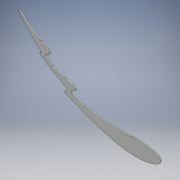
# Autodesk Inventor part: bracket
Saved by Autodesk Inventor 2018.2 (Build 222227000, 227)
## iProperties
Created: 2018-03-14
Part Number: bracket
Material: 一般
Document SubType Name: Modeling
Designer: ku_sk
Density: 1 g/cm^3
Appearance: 既定
Author: ku_sk
Autodesk Inventor part; units mm, degrees
ref_plane "YZ Plane" through (0, 0, 0) normal (1, 0, 0) x (0, 1, 0)
ref_plane "XZ Plane" through (0, 0, 0) normal (0, 1, 0) x (-1, 0, 0)
ref_plane "XY Plane" through (0, 0, 0) normal (0, 0, 1) x (1, 0, 0)
sketch "スケッチ1" plane through (0, 0, 0) normal (0, 1, 0) x (-1, 0, 0)
  arc A0 (352.9404, 45.4012) -> (350.2664, 52.9074) centre (351.268, 49.0348) ccw projected
  arc A1 (196.042, -12.8796) -> (352.9404, 45.4012) centre (-109.7603, 1050.7077) ccw projected
  arc A2 (150.312, -24.5744) -> (196.042, -12.8796) centre (-24.3171, 753.5344) ccw projected
  arc A3 (62.5903, -32.1265) -> (150.312, -24.5744) centre (78.6271, 294.8376) ccw projected
  arc A4 (7.8921, -21.3368) -> (62.5903, -32.1265) centre (71.9931, 159.5809) ccw projected
  arc A5 (-9.4003, -11.6891) -> (7.8921, -21.3368) centre (27.6212, 34.3463) ccw projected
  arc A6 (-8.119, 12.6128) -> (-9.4003, -11.6891) centre (0, 0) ccw projected
  arc A7 (11.7348, 20.8189) -> (-8.119, 12.6128) centre (24.3569, -37.8384) ccw projected
  arc A8 (90.7942, 27.108) -> (11.7348, 20.8189) centre (74.8452, -272.4677) ccw projected
  arc A9 (90.7942, 27.108) -> (95.7842, 26.8528) centre (154.5899, 1225.411) ccw projected
  arc A10 (95.7842, 26.8528) -> (350.2664, 52.9074) centre (137.4382, 875.8316) ccw projected
  arc A11 (451.6654, 129.0808) -> (449.8552, 131.7041) centre (450.6431, 130.3115) ccw projected
  arc A12 (397.0782, 90.3195) -> (451.6654, 129.0808) centre (168.8146, 469.5991) ccw projected
  arc A13 (380.6202, 81.0666) -> (397.0782, 90.3195) centre (232.593, 363.6259) ccw projected
  arc A14 (347.509, 69.0671) -> (380.6202, 81.0666) centre (319.8553, 197.0566) ccw projected
  arc A15 (325.2582, 67.5731) -> (347.509, 69.0671) centre (331.295, 144.1106) ccw projected
  arc A16 (317.5781, 69.5105) -> (325.2582, 67.5731) centre (327.1162, 91.13) ccw projected
  arc A17 (315.5573, 79.0327) -> (317.5781, 69.5105) centre (320, 75) ccw projected
  arc A18 (322.3786, 84.2587) -> (315.5573, 79.0327) centre (333.3281, 62.902) ccw projected
  arc A19 (352.2737, 94.8734) -> (322.3786, 84.2587) centre (377.1259, -22.5249) ccw projected
  arc A20 (352.2737, 94.8734) -> (354.2282, 95.2914) centre (252.865, 564.4668) ccw projected
  arc A21 (354.2282, 95.2914) -> (449.8552, 131.7041) centre (282.4293, 427.624) ccw projected
  arc A22 (533.1819, 231.3155) -> (533.0183, 233.3599) centre (531.8758, 232.2398) ccw projected
  arc A23 (490.4869, 179.7468) -> (533.1819, 231.3155) centre (171.8364, 487.0238) ccw projected
  arc A24 (476.9845, 166.5496) -> (490.4869, 179.7468) centre (260.8694, 401.1686) ccw projected
  arc A25 (448.1072, 146.3891) -> (476.9845, 166.5496) centre (388.2697, 262.8602) ccw projected
  arc A26 (427.0013, 139.1871) -> (448.1072, 146.3891) centre (413.023, 214.679) ccw projected
  arc A27 (419.0814, 139.0707) -> (427.0013, 139.1871) centre (422.699, 162.4222) ccw projected
  arc A28 (414.665, 147.7454) -> (419.0814, 139.0707) centre (420, 145) ccw projected
  arc A29 (419.9012, 154.5588) -> (414.665, 147.7454) centre (436.0051, 136.7638) ccw projected
  arc A30 (446.0304, 172.5493) -> (419.9012, 154.5588) centre (500.4207, 65.5835) ccw projected
  arc A31 (446.0304, 172.5493) -> (447.8101, 173.4589) centre (228.4693, 600.4128) ccw projected
  arc A32 (447.8101, 173.4589) -> (530.4702, 233.1021) centre (292.4437, 475.8846) ccw projected
  line L0 (530.4702, 233.1021) -> (525.5697, 238.1005) projected
  line L1 (525.5697, 238.1005) -> (526.9978, 239.5007) projected
  line L2 (526.9978, 239.5007) -> (533.0183, 233.3599) projected
  arc A33 (530.4702, 233.1021) -> (530.7544, 233.381) centre (292.4437, 475.8846) ccw
  arc A34 (533.0183, 233.3599) -> (530.7544, 233.381) centre (531.8758, 232.2398) ccw
  line L3 (317.5781, 69.5105) -> (338.9513, 60.0811)
  line L4 (338.9513, 60.0811) -> (283.0095, 38.3896)
  line L5 (380.6202, 81.0666) -> (345.1511, 62.485)
  line L6 (345.1511, 62.485) -> (354.3249, 51.6146)
  line L7 (419.0814, 139.0707) -> (435.7934, 136.4817)
  line L8 (435.7934, 136.4817) -> (395.4422, 106.9558)
  line L9 (476.9845, 166.5496) -> (443.1114, 135.348)
  line L10 (443.1114, 135.348) -> (451.2836, 131.7777)
  point P0 (0, 0)
  dimension "d2" = 45
  dimension "d3" = 45
  dimension "d4" = 60
  dimension "d5" = 50
  constraints: 16 end point, 8 point on circle, 7 tangent, 2 centre point, 2 concentric, 2 point on line
  measures "d2" angle of L4 L3
  measures "d3" angle of L8 L7
  measures "d4" distance of L3.end L4.end
  measures "d5" distance of L7.end L8.end
extrude "押し出し1" add sketch "スケッチ1" along normal mid plane 4 contours A1 A2 A3 A4 A5 A6 A7 A8 A9 A10 A0 | A0 A10 L4 L3 A16 A15 A14 L5 L6 | A14 A15 A16 A17 A18 A19 A20 A21 A11 A12 A13 | A11 A21 L8 L7 A27 A26 A25 L9 L10 | A25 A26 A27 A28 A29 A30 A31 A32 A33 A34 A22 A23 A24
fillet "フィレット1" radius 4 2 edges at (-338.9513, 0, 60.0811) (-435.7934, 0, 136.4817)
fillet "フィレット1" radius 3 2 edges at (-443.1114, 0, 135.348) (-345.1511, 0, 62.485)
fillet "フィレット1" radius 50 2 edges at (-395.4422, 0, 106.9558) (-283.0095, 0, 38.3896)
